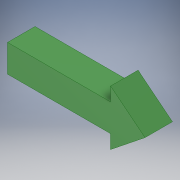
# Autodesk Inventor part: ArrowUp
Saved by Autodesk Inventor 2018.2 (Build 222227000, 227)
## iProperties
Created: 2018-04-16
Part Number: ArrowUp
Material: Generisch
Document SubType Name: Modeling
Designer: Nick Koch
Density: 1 g/cm^3
Appearance: Glatt - waldgrün
Author: Nick Koch
Autodesk Inventor part; units mm, degrees
ref_plane "YZ Plane" through (0, 0, 0) normal (1, 0, 0) x (0, 1, 0)
ref_plane "XZ Plane" through (0, 0, 0) normal (0, 1, 0) x (-1, 0, 0)
ref_plane "XY Plane" through (0, 0, 0) normal (0, 0, 1) x (1, 0, 0)
sketch "Skizze1" plane through (0, 0, 0) normal (0, 0, 1) x (1, 0, 0)
  line L0 (0, 0) -> (15, 0)
  line L1 (15, 0) -> (15, 4)
  line L2 (15, 4) -> (0, 4)
  line L3 (0, 4) -> (0, 0)
  dimension "d0" = 15
  dimension "d1" = 4
  constraints: 8 end point, 2 parallel, 1 horizontal, 1 perpendicular
  measures "d0" distance of L2.end L1.end
  measures "d1" distance of L1.end L0.end
extrude "Extrusion1" add sketch "Skizze1" along normal blind 4
sketch "Skizze2" plane through (0, 0, 0) normal (0, -1, 0) x (1, 0, 0)
  line L0 (15, 0) -> (15, 4) projected
  line L1 (15, 2) -> (15, 6)
  line L2 (15, 6) -> (15, -2)
  line L3 (15, 2) -> (20, 2)
  line L4 (20, 2) -> (15, -2)
  line L5 (15, 6) -> (20, 2)
  point P0 (0, 0)
  dimension "d4" = 4
  dimension "d5" = 8
  dimension "d6" = 5
  constraints: 10 end point, 2 point on line, 1 horizontal, 1 midpoint
  measures "d4" distance of L1.start L1.end
  measures "d5" distance of L1.end L2.end
  measures "d6" distance of L1.start L3.end
extrude "Extrusion2" add sketch "Skizze2" against normal blind 4
